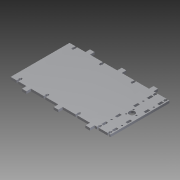
# Autodesk Inventor part: pieza central base inferior
Saved by Autodesk Inventor 2012 SP1 (Build 160190100, 190)
## iProperties
Created: 2014-12-27
Part Number: pieza central base inferior
Material: Default
Document SubType Name: Modeling
Designer: PRINCIPAL
Density: 1 g/cm^3
Author: PRINCIPAL
Autodesk Inventor part; units mm, degrees
ref_plane "YZ Plane" through (0, 0, 0) normal (1, 0, 0) x (0, 1, 0)
ref_plane "XZ Plane" through (0, 0, 0) normal (0, 1, 0) x (-1, 0, 0)
ref_plane "XY Plane" through (0, 0, 0) normal (0, 0, 1) x (1, 0, 0)
sketch "Boceto1" plane through (0, 0, 0) normal (0, 0, 1) x (1, 0, 0)
  line L0 (215, 0) -> (185, 0)
  line L1 (185, 0) -> (185, 10)
  line L2 (185, 10) -> (175, 10)
  line L3 (175, 10) -> (175, 0)
  line L4 (175, 0) -> (115, 0)
  line L5 (115, 0) -> (115, 10)
  line L6 (115, 10) -> (105, 10)
  line L7 (105, 10) -> (105, 0)
  line L8 (105, 0) -> (45, 0)
  line L9 (45, 0) -> (45, 10)
  line L10 (45, 10) -> (35, 10)
  line L11 (35, 10) -> (35, 0)
  line L12 (35, 0) -> (0, 0)
  line L13 (0, 0) -> (0, -130)
  line L14 (0, -130) -> (35, -130)
  line L15 (35, -130) -> (35, -140)
  line L16 (35, -140) -> (45, -140)
  line L17 (45, -140) -> (45, -130)
  line L18 (45, -130) -> (105, -130)
  line L19 (105, -130) -> (105, -140)
  line L20 (105, -140) -> (115, -140)
  line L21 (115, -140) -> (115, -130)
  line L22 (115, -130) -> (175, -130)
  line L23 (175, -130) -> (175, -140)
  line L24 (175, -140) -> (185, -140)
  line L25 (196.8872, -130) -> (215, -130)
  line L26 (185, -140) -> (185, -130)
  line L27 (185, -130) -> (196.8872, -130)
  line L28 (220, 0) -> (220, -130)
  line L29 (215, 0) -> (220, 0)
  line L30 (215, -130) -> (220, -130)
  dimension "d4" = 60
  dimension "d5" = 60
  dimension "d7" = 10
  dimension "d8" = 60
  dimension "d10" = 60
  dimension "d12" = 10
  dimension "d13" = 10
  dimension "d15" = 10
  dimension "d16" = 10
  dimension "d17" = 10
  dimension "d34" = 10
  dimension "d35" = 10
  dimension "d36" = 10
  dimension "d37" = 10
  dimension "d38" = 10
  dimension "d39" = 10
  dimension "d40" = 10
  dimension "d41" = 10
  dimension "d42" = 10
  dimension "d43" = 10
  dimension "d44" = 10
  dimension "d45" = 10
  dimension "d46" = 130
  constraints: 62 end point, 3 perpendicular, 1 parallel, 1 point on line
  measures "d4" distance between parallel lines of L19 L17
  measures "d5" distance between parallel lines of L23 L21
  measures "d7" distance between parallel lines of L23 L26
  measures "d8" distance between parallel lines of L7 L9
  measures "d10" distance between parallel lines of L3 L5
  measures "d12" distance between parallel lines of L21 L19
  measures "d13" distance between parallel lines of L17 L15
  measures "d15" distance between parallel lines of L1 L3
  measures "d16" distance between parallel lines of L5 L7
  measures "d17" distance between parallel lines of L9 L11
  measures "d34" distance from line of L8 L9.end
  measures "d35" distance from line of L4 L5.end
  measures "d36" distance from line of L0 L1.end
  measures "d37" distance from line of L10.end L12
  measures "d38" distance between parallel lines of L8 L6
  measures "d39" distance between parallel lines of L4 L2
  measures "d40" distance between parallel lines of L14 L16
  measures "d41" distance between parallel lines of L18 L16
  measures "d42" distance between parallel lines of L18 L20
  measures "d43" distance between parallel lines of L20 L22
  measures "d44" distance between parallel lines of L22 L24
  measures "d45" distance from line of L24.end L27
  measures "d46" distance between parallel lines of L14 L12
extrude "Extrusión1" add sketch "Boceto1" along normal blind 5
sketch "Boceto2" plane through (0, 0, 5) normal (0, 0, 1) x (1, 0, 0)
  circle A0 centre (197.85, -73.2272) radius 1.75
  circle A1 centre (197.85, -56.7728) radius 1.75
  circle A2 centre (212.1, -65) radius 1.75
  circle A3 centre (202.6, -65) radius 6.35
  line L0 (220, -130) -> (185, -130) projected
  dimension "d19" = 3.5
  dimension "d20" = 3.5
  dimension "d21" = 3.5
  dimension "d22" = 14.25
  dimension "d23" = 16.4545
  dimension "d27" = 12.7
  dimension "d31" = 65
  dimension "d32" = 65
  constraints: 4 centre point, 3 coincident
  measures "d19" diameter of A0
  measures "d20" diameter of A1
  measures "d21" diameter of A2
  measures "d22" horizontal distance of A1.centre A2.centre
  measures "d23" distance of A1.centre A0.centre
  measures "d27" diameter of A3
  measures "d31" distance from line of L0 A2.centre
  measures "d32" distance from line of L0 A3.centre
extrude "Extrusión2" cut sketch "Boceto2" against normal blind 5
sketch "Boceto3" plane through (0, 0, 5) normal (0, 0, 1) x (1, 0, 0)
  line L0 (220, -130) -> (185, -130) projected
  line L1 (220, 0) -> (220, -130) projected
  line L2 (185, 0) -> (220, 0) projected
  line L3 (213, -10) -> (218, -10)
  line L4 (218, -10) -> (218, -20)
  line L5 (218, -20) -> (213, -20)
  line L6 (213, -20) -> (213, -10)
  line L7 (213, -110) -> (218, -110)
  line L8 (218, -110) -> (218, -120)
  line L9 (218, -120) -> (213, -120)
  line L10 (213, -120) -> (213, -110)
  line L11 (213, -80) -> (218, -80)
  line L12 (218, -80) -> (218, -90)
  line L13 (218, -90) -> (213, -90)
  line L14 (213, -90) -> (213, -80)
  line L15 (213, -40) -> (218, -40)
  line L16 (218, -40) -> (218, -50)
  line L17 (218, -50) -> (213, -50)
  line L18 (213, -50) -> (213, -40)
  circle A0 centre (215.5, -30) radius 1.75
  circle A1 centre (215.5, -100) radius 1.75
  line L19 (190, -10) -> (195, -10)
  line L20 (195, -10) -> (195, -20)
  line L21 (195, -20) -> (190, -20)
  line L22 (190, -20) -> (190, -10)
  line L23 (190, -110) -> (195, -110)
  line L24 (195, -110) -> (195, -120)
  line L25 (195, -120) -> (190, -120)
  line L26 (190, -120) -> (190, -110)
  line L27 (190, -80) -> (195, -80)
  line L28 (195, -80) -> (195, -90)
  line L29 (195, -90) -> (190, -90)
  line L30 (190, -90) -> (190, -80)
  line L31 (190, -40) -> (195, -40)
  line L32 (195, -40) -> (195, -50)
  line L33 (195, -50) -> (190, -50)
  line L34 (190, -50) -> (190, -40)
  circle A2 centre (192.5, -30) radius 1.75
  circle A3 centre (192.5, -100) radius 1.75
  dimension "d48" = 3.5
  dimension "d49" = 3.5
  dimension "d50" = 5
  dimension "d51" = 10
  dimension "d52" = 10
  dimension "d53" = 5
  dimension "d54" = 10
  dimension "d55" = 5
  dimension "d56" = 10
  dimension "d57" = 5
  dimension "d58" = 2
  dimension "d59" = 2
  dimension "d60" = 2
  dimension "d61" = 2
  dimension "d62" = 10
  dimension "d63" = 20
  dimension "d64" = 10
  dimension "d65" = 20
  dimension "d66" = 4.5
  dimension "d67" = 10
  dimension "d68" = 4.5
  dimension "d69" = 10
  dimension "d72" = 3.5
  dimension "d73" = 3.5
  dimension "d74" = 5
  dimension "d75" = 10
  dimension "d76" = 10
  dimension "d77" = 5
  dimension "d78" = 10
  dimension "d79" = 5
  dimension "d80" = 10
  dimension "d81" = 5
  dimension "d82" = 20
  dimension "d83" = 20
  dimension "d84" = 10
  dimension "d85" = 10
  dimension "d86" = 23
  dimension "d87" = 23
  dimension "d88" = 23
  dimension "d89" = 23
  dimension "d90" = 2.5
  constraints: 64 end point, 16 parallel, 8 horizontal, 8 perpendicular, 4 centre point
  measures "d48" diameter of A0
  measures "d49" diameter of A1
  measures "d50" distance between parallel lines of L8 L10
  measures "d51" distance between parallel lines of L7 L9
  measures "d52" distance between parallel lines of L11 L13
  measures "d53" distance between parallel lines of L12 L14
  measures "d54" distance between parallel lines of L17 L15
  measures "d55" distance between parallel lines of L16 L18
  measures "d56" distance between parallel lines of L3 L5
  measures "d57" distance between parallel lines of L4 L6
  measures "d58" distance between parallel lines of L1 L4
  measures "d59" distance between parallel lines of L1 L16
  measures "d60" distance between parallel lines of L1 L12
  measures "d61" distance between parallel lines of L1 L8
  measures "d62" distance between parallel lines of L0 L9
  measures "d63" distance between parallel lines of L13 L7
  measures "d64" distance between parallel lines of L2 L3
  measures "d65" distance between parallel lines of L15 L5
  measures "d66" distance from line of L1 A0.centre
  measures "d67" distance from line of A0.centre L15
  measures "d68" distance from line of L1 A1.centre
  measures "d69" distance from line of A1.centre L7
  measures "d72" diameter of A2
  measures "d73" diameter of A3
  measures "d74" distance between parallel lines of L24 L26
  measures "d75" distance between parallel lines of L23 L25
  measures "d76" distance between parallel lines of L27 L29
  measures "d77" distance between parallel lines of L28 L30
  measures "d78" distance between parallel lines of L33 L31
  measures "d79" distance between parallel lines of L32 L34
  measures "d80" distance between parallel lines of L19 L21
  measures "d81" distance between parallel lines of L20 L22
  measures "d82" distance between parallel lines of L29 L23
  measures "d83" distance between parallel lines of L31 L21
  measures "d84" distance from line of A2.centre L31
  measures "d85" distance from line of A3.centre L23
  measures "d86" distance of L29.end L13.end
  measures "d87" distance between parallel lines of L10 L26
  measures "d88" distance between parallel lines of L6 L22
  measures "d89" distance between parallel lines of L18 L34
  measures "d90" distance from line of L24 A3.centre
extrude "Extrusión4" cut sketch "Boceto3" against normal blind 10
sketch "Boceto4" plane through (0, 0, 5) normal (0, 0, 1) x (1, 0, 0)
  line L0 (190.6018, -132.1796) -> (190.6018, -127.2682)
  line L1 (194.1018, -132.1796) -> (190.6018, -132.1796)
  line L2 (194.1018, -127.2682) -> (194.1018, -132.1796)
  line L3 (190.6018, -127.2682) -> (189.6018, -127.2682)
  line L4 (189.6018, -124.8682) -> (190.6018, -124.8682)
  line L5 (190.6018, -124.8682) -> (190.6018, -122.0942)
  line L6 (194.1018, -122.0942) -> (194.1018, -124.8682)
  line L7 (195.1018, -127.2682) -> (194.1018, -127.2682)
  line L8 (195.1018, -124.8682) -> (195.1018, -127.2682)
  line L9 (194.1018, -124.8682) -> (195.1018, -124.8682)
  line L10 (194.1018, -122.0942) -> (190.6018, -122.0942)
  line L11 (189.6018, -127.2682) -> (189.6018, -124.8682)
  line L12 (213.75, -132.1796) -> (213.75, -127.2682)
  line L13 (217.25, -132.1796) -> (213.75, -132.1796)
  line L14 (217.25, -127.2682) -> (217.25, -132.1796)
  line L15 (213.75, -127.2682) -> (212.75, -127.2682)
  line L16 (212.75, -124.8682) -> (213.75, -124.8682)
  line L17 (213.75, -124.8682) -> (213.75, -122.0942)
  line L18 (217.25, -122.0942) -> (217.25, -124.8682)
  line L19 (218.25, -127.2682) -> (217.25, -127.2682)
  line L20 (218.25, -124.8682) -> (218.25, -127.2682)
  line L21 (217.25, -124.8682) -> (218.25, -124.8682)
  line L22 (217.25, -122.0942) -> (213.75, -122.0942)
  line L23 (212.75, -127.2682) -> (212.75, -124.8682)
  line L24 (143.3616, -131.1704) -> (143.3616, -126.2591)
  line L25 (146.8616, -131.1704) -> (143.3616, -131.1704)
  line L26 (146.8616, -126.2591) -> (146.8616, -131.1704)
  line L27 (143.3616, -126.2591) -> (142.3616, -126.2591)
  line L28 (142.3616, -123.8591) -> (143.3616, -123.8591)
  line L29 (143.3616, -123.8591) -> (143.3616, -121.085)
  line L30 (146.8616, -121.085) -> (146.8616, -123.8591)
  line L31 (147.8616, -126.2591) -> (146.8616, -126.2591)
  line L32 (147.8616, -123.8591) -> (147.8616, -126.2591)
  line L33 (146.8616, -123.8591) -> (147.8616, -123.8591)
  line L34 (146.8616, -121.085) -> (143.3616, -121.085)
  line L35 (142.3616, -126.2591) -> (142.3616, -123.8591)
  line L36 (73.2599, -131.1704) -> (73.2599, -126.2591)
  line L37 (76.7599, -131.1704) -> (73.2599, -131.1704)
  line L38 (76.7599, -126.2591) -> (76.7599, -131.1704)
  line L39 (73.2599, -126.2591) -> (72.2599, -126.2591)
  line L40 (72.2599, -123.8591) -> (73.2599, -123.8591)
  line L41 (73.2599, -123.8591) -> (73.2599, -121.085)
  line L42 (76.7599, -121.085) -> (76.7599, -123.8591)
  line L43 (77.7599, -126.2591) -> (76.7599, -126.2591)
  line L44 (77.7599, -123.8591) -> (77.7599, -126.2591)
  line L45 (76.7599, -123.8591) -> (77.7599, -123.8591)
  line L46 (76.7599, -121.085) -> (73.2599, -121.085)
  line L47 (72.2599, -126.2591) -> (72.2599, -123.8591)
  line L48 (13.2369, -130) -> (13.2369, -125.0887)
  line L49 (16.7369, -130) -> (13.2369, -130)
  line L50 (16.7369, -125.0887) -> (16.7369, -130)
  line L51 (13.2369, -125.0887) -> (12.2369, -125.0887)
  line L52 (12.2369, -122.6887) -> (13.2369, -122.6887)
  line L53 (13.2369, -122.6887) -> (13.2369, -119.9146)
  line L54 (16.7369, -119.9146) -> (16.7369, -122.6887)
  line L55 (17.7369, -125.0887) -> (16.7369, -125.0887)
  line L56 (17.7369, -122.6887) -> (17.7369, -125.0887)
  line L57 (16.7369, -122.6887) -> (17.7369, -122.6887)
  line L58 (16.7369, -119.9146) -> (13.2369, -119.9146)
  line L59 (12.2369, -125.0887) -> (12.2369, -122.6887)
  line L60 (217.1781, 2.6307) -> (217.1781, -2.2806)
  line L61 (213.6781, 2.6307) -> (217.1781, 2.6307)
  line L62 (213.6781, -2.2806) -> (213.6781, 2.6307)
  line L63 (217.1781, -2.2806) -> (218.1781, -2.2806)
  line L64 (218.1781, -4.6806) -> (217.1781, -4.6806)
  line L65 (217.1781, -4.6806) -> (217.1781, -7.4546)
  line L66 (213.6781, -7.4546) -> (213.6781, -4.6806)
  line L67 (212.6781, -2.2806) -> (213.6781, -2.2806)
  line L68 (212.6781, -4.6806) -> (212.6781, -2.2806)
  line L69 (213.6781, -4.6806) -> (212.6781, -4.6806)
  line L70 (213.6781, -7.4546) -> (217.1781, -7.4546)
  line L71 (218.1781, -2.2806) -> (218.1781, -4.6806)
  line L72 (194.1018, 2.6307) -> (194.1018, -2.2806)
  line L73 (190.6018, 2.6307) -> (194.1018, 2.6307)
  line L74 (190.6018, -2.2806) -> (190.6018, 2.6307)
  line L75 (194.1018, -2.2806) -> (195.1018, -2.2806)
  line L76 (195.1018, -4.6806) -> (194.1018, -4.6806)
  line L77 (194.1018, -4.6806) -> (194.1018, -7.4546)
  line L78 (190.6018, -7.4546) -> (190.6018, -4.6806)
  line L79 (189.6018, -2.2806) -> (190.6018, -2.2806)
  line L80 (189.6018, -4.6806) -> (189.6018, -2.2806)
  line L81 (190.6018, -4.6806) -> (189.6018, -4.6806)
  line L82 (190.6018, -7.4546) -> (194.1018, -7.4546)
  line L83 (195.1018, -2.2806) -> (195.1018, -4.6806)
  line L84 (146.6908, 1.0321) -> (146.6908, -3.8792)
  line L85 (143.1908, 1.0321) -> (146.6908, 1.0321)
  line L86 (143.1908, -3.8792) -> (143.1908, 1.0321)
  line L87 (146.6908, -3.8792) -> (147.6908, -3.8792)
  line L88 (147.6908, -6.2792) -> (146.6908, -6.2792)
  line L89 (146.6908, -6.2792) -> (146.6908, -9.0532)
  line L90 (143.1908, -9.0532) -> (143.1908, -6.2792)
  line L91 (142.1908, -3.8792) -> (143.1908, -3.8792)
  line L92 (142.1908, -6.2792) -> (142.1908, -3.8792)
  line L93 (143.1908, -6.2792) -> (142.1908, -6.2792)
  line L94 (143.1908, -9.0532) -> (146.6908, -9.0532)
  line L95 (147.6908, -3.8792) -> (147.6908, -6.2792)
  line L96 (76.8096, 1.0321) -> (76.8096, -3.8792)
  line L97 (73.3096, 1.0321) -> (76.8096, 1.0321)
  line L98 (73.3096, -3.8792) -> (73.3096, 1.0321)
  line L99 (76.8096, -3.8792) -> (77.8096, -3.8792)
  line L100 (77.8096, -6.2792) -> (76.8096, -6.2792)
  line L101 (76.8096, -6.2792) -> (76.8096, -9.0532)
  line L102 (73.3096, -9.0532) -> (73.3096, -6.2792)
  line L103 (72.3096, -3.8792) -> (73.3096, -3.8792)
  line L104 (72.3096, -6.2792) -> (72.3096, -3.8792)
  line L105 (73.3096, -6.2792) -> (72.3096, -6.2792)
  line L106 (73.3096, -9.0532) -> (76.8096, -9.0532)
  line L107 (77.8096, -3.8792) -> (77.8096, -6.2792)
  line L108 (16.7707, 0.7543) -> (16.7707, -4.157)
  line L109 (13.2707, 0.7543) -> (16.7707, 0.7543)
  line L110 (13.2707, -4.157) -> (13.2707, 0.7543)
  line L111 (16.7707, -4.157) -> (17.7707, -4.157)
  line L112 (17.7707, -6.557) -> (16.7707, -6.557)
  line L113 (16.7707, -6.557) -> (16.7707, -9.331)
  line L114 (13.2707, -9.331) -> (13.2707, -6.557)
  line L115 (12.2707, -4.157) -> (13.2707, -4.157)
  line L116 (12.2707, -6.557) -> (12.2707, -4.157)
  line L117 (13.2707, -6.557) -> (12.2707, -6.557)
  line L118 (13.2707, -9.331) -> (16.7707, -9.331)
  line L119 (17.7707, -4.157) -> (17.7707, -6.557)
  line L120 (220, 0) -> (220, -130) projected
  line L121 (115, 0) -> (175, 0) projected
  line L122 (185, -130) -> (185, -140) projected
  line L123 (145, 0) -> (145, -149.5904)
  line L124 (105, -140) -> (105, -130) projected
  line L125 (185, -140) -> (175, -140) projected
  line L126 (75, 12.0285) -> (75, -142.1824)
  point P0 (0, 0)
  dimension "d93" = 3.5
  dimension "d94" = 3.5
  dimension "d95" = 3.5
  dimension "d96" = 3.5
  dimension "d97" = 3.5
  dimension "d98" = 3.5
  dimension "d99" = 3.5
  dimension "d100" = 3.5
  dimension "d101" = 3.5
  dimension "d102" = 3.5
  dimension "d108" = 75
  dimension "d109" = 13.2707
  dimension "d110" = 30
  constraints: 244 end point, 1 midpoint, 1 parallel, 1 perpendicular
  measures "d93" distance between parallel lines of L5 L6
  measures "d94" distance between parallel lines of L17 L18
  measures "d95" distance between parallel lines of L29 L30
  measures "d96" distance between parallel lines of L41 L42
  measures "d97" distance between parallel lines of L53 L54
  measures "d98" distance between parallel lines of L65 L66
  measures "d99" distance between parallel lines of L77 L78
  measures "d100" distance between parallel lines of L89 L90
  measures "d101" distance between parallel lines of L101 L102
  measures "d102" distance between parallel lines of L113 L114
  measures "d108" distance between parallel lines of L120 L123
  measures "d109" horizontal distance of L110.end point (0, 0)
  measures "d110" distance between parallel lines of L124 L126
extrude "Extrusión5" cut sketch "Boceto4" against normal blind 10
